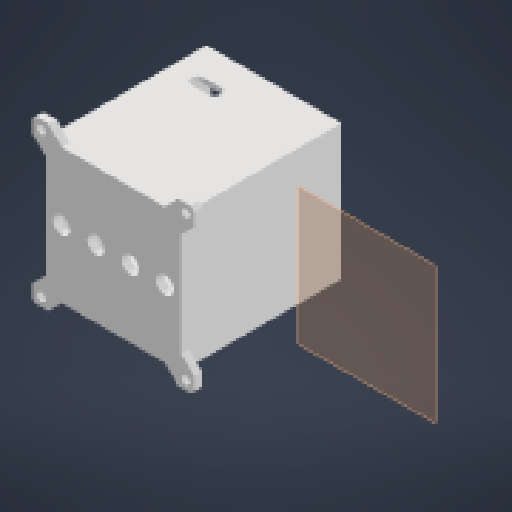
# Autodesk Inventor part: casing_1x1_lvl3
Saved by Autodesk Inventor 2024 (Build 280153000, 153)
## iProperties
Created: 2026-04-07
Part Number: casing_1x1_lvl3
Material: Generic
Document SubType Name: Modeling
Designer: schar
Density: 1 g/cm^3
Appearance: Default
Author: schar
Autodesk Inventor part; units mm, degrees
ref_plane "YZ Plane" through (0, 0, 0) normal (1, 0, 0) x (0, 1, 0)
ref_plane "XZ Plane" through (0, 0, 0) normal (0, 1, 0) x (-1, 0, 0)
ref_plane "XY Plane" through (0, 0, 0) normal (0, 0, 1) x (1, 0, 0)
sketch "Sketch1" plane through (0, 0, 0) normal (0, 0, 1) x (1, 0, 0)
  line L0 (51.6317, -54.9773) -> (91.6317, -54.9773) projected
  line L1 (94.6317, -57.9773) -> (94.5909, -98.4705) projected
  line L2 (48.6317, -97.9773) -> (48.6317, -57.9773) projected
  line L3 (91.6317, -100.9773) -> (51.6317, -100.9773) projected
  line L4 (48.6317, -77.9773) -> (94.6113, -78.2239)
  line L5 (71.6317, -54.9773) -> (71.6317, -100.9773)
  line L6 (48.5522, -54.8773) -> (94.7112, -54.8773)
  line L7 (94.7112, -54.8773) -> (94.7112, -101.0773)
  line L8 (94.7112, -101.0773) -> (48.5522, -101.0773)
  line L9 (48.5522, -101.0773) -> (48.5522, -54.8773)
  line L10 (48.5522, -54.8773) -> (94.7112, -101.0773) construction
  line L11 (94.7112, -54.8773) -> (48.5522, -101.0773) construction
  line L12 (46.6317, -52.9773) -> (96.6317, -52.9773)
  line L13 (96.6317, -52.9773) -> (96.6317, -102.9773)
  line L14 (96.6317, -102.9773) -> (46.6317, -102.9773)
  line L15 (46.6317, -102.9773) -> (46.6317, -52.9773)
  line L16 (46.6317, -52.9773) -> (96.6317, -102.9773) construction
  line L17 (96.6317, -52.9773) -> (46.6317, -102.9773) construction
  line L18 (36.6317, -42.9773) -> (106.6317, -42.9773)
  line L19 (106.6317, -42.9773) -> (106.6317, -112.9773)
  line L20 (106.6317, -112.9773) -> (36.6317, -112.9773)
  line L21 (36.6317, -112.9773) -> (36.6317, -42.9773)
  line L22 (36.6317, -42.9773) -> (106.6317, -112.9773) construction
  line L23 (106.6317, -42.9773) -> (36.6317, -112.9773) construction
  point P0 (0, 0)
  point P1 (71.6317, -77.9773)
  dimension "d0" = 46.159
  dimension "d1" = 46.2
  dimension "d2" = 50
  dimension "d3" = 50
  dimension "d4" = 70
  dimension "d5" = 70
  constraints: 40 end point, 11 midpoint, 6 parallel, 3 horizontal, 3 perpendicular
  measures "d0" distance of L7.end L8.end
  measures "d1" distance of L6.end L7.end
  measures "d2" distance of L13.end L14.end
  measures "d3" distance of L12.end L13.end
  measures "d4" distance of L19.end L20.end
  measures "d5" distance of L18.end L19.end
extrude "Extrusion1" add sketch "Sketch1" along normal blind 40 and the other way blind 30 contours L12 L13 L14 L15
ref_plane "Work Plane1" through (0, 0, 0) normal (0, 0, 1) x (1, 0, 0)
sketch "Sketch2" plane through (0, 0, 0) normal (0, 0, 1) x (1, 0, 0)
  arc A0 (94.6317, -57.9773) -> (91.6317, -54.9773) centre (91.6317, -57.9773) ccw projected
  line L0 (51.6317, -54.9773) -> (91.6317, -54.9773) projected
  arc A1 (51.6317, -54.9773) -> (48.6317, -57.9773) centre (51.6317, -57.9773) ccw projected
  line L1 (48.6317, -97.9773) -> (48.6317, -57.9773) projected
  arc A2 (48.6317, -97.9773) -> (51.6317, -100.9773) centre (51.6317, -97.9773) ccw projected
  line L2 (91.6317, -100.9773) -> (51.6317, -100.9773) projected
  arc A3 (91.6317, -100.9773) -> (94.5909, -98.4705) centre (91.6317, -97.9773) ccw projected
  line L3 (94.6317, -57.9773) -> (94.5909, -98.4705) projected
  circle A4 centre (51.6317, -97.9773) radius 1.1 projected
  circle A5 centre (56.1317, -83.4773) radius 1.725 projected
  circle A6 centre (62.4817, -82.2073) radius 0.45 projected
  circle A7 centre (65.0217, -80.9373) radius 0.45 projected
  circle A8 centre (62.4817, -79.6673) radius 0.45 projected
  circle A9 centre (65.0217, -78.3973) radius 0.45 projected
  circle A10 centre (72.1317, -96.7573) radius 0.5 projected
  circle A11 centre (72.1317, -94.2173) radius 0.5 projected
  circle A12 centre (72.1317, -91.6773) radius 0.5 projected
  circle A13 centre (72.1317, -89.1373) radius 0.5 projected
  circle A14 centre (79.1317, -89.9898) radius 0.4 projected
  circle A15 centre (91.6317, -97.9773) radius 1.1 projected
  circle A16 centre (86.7517, -89.9898) radius 0.4 projected
  circle A17 centre (72.1317, -86.5973) radius 0.5 projected
  circle A18 centre (72.1317, -84.0573) radius 0.5 projected
  circle A19 centre (72.1317, -81.5173) radius 0.5 projected
  circle A20 centre (72.1317, -78.9773) radius 0.5 projected
  circle A21 centre (78.5917, -81.7473) radius 0.45 projected
  circle A22 centre (78.5917, -79.2073) radius 0.45 projected
  circle A23 centre (81.1317, -80.4773) radius 0.45 projected
  circle A24 centre (87.4817, -83.0173) radius 1.725 projected
  circle A25 centre (56.1317, -72.0473) radius 1.725 projected
  circle A26 centre (62.4817, -77.1273) radius 0.45 projected
  circle A27 centre (65.0217, -75.8573) radius 0.45 projected
  circle A28 centre (62.4817, -74.5873) radius 0.45 projected
  circle A29 centre (65.0217, -73.3173) radius 0.45 projected
  arc A30 (55.0117, -62.6123) -> (55.6117, -62.6123) centre (55.3117, -62.6123) ccw projected
  line L4 (55.0117, -62.6123) -> (55.0117, -61.5123) projected
  arc A31 (55.6117, -61.5123) -> (55.0117, -61.5123) centre (55.3117, -61.5123) ccw projected
  line L5 (55.6117, -61.5123) -> (55.6117, -62.6123) projected
  circle A32 centre (51.6317, -57.9773) radius 1.1 projected
  arc A33 (55.0117, -58.1823) -> (55.6117, -58.1823) centre (55.3117, -58.1823) ccw projected
  line L6 (55.0117, -58.1823) -> (55.0117, -57.5823) projected
  arc A34 (55.6117, -57.5823) -> (55.0117, -57.5823) centre (55.3117, -57.5823) ccw projected
  line L7 (55.6117, -57.5823) -> (55.6117, -58.1823) projected
  circle A35 centre (56.7417, -61.5323) radius 0.325 projected
  circle A36 centre (62.5217, -61.5323) radius 0.325 projected
  arc A37 (63.6517, -62.6123) -> (64.2517, -62.6123) centre (63.9517, -62.6123) ccw projected
  line L8 (63.6517, -62.6123) -> (63.6517, -61.5123) projected
  arc A38 (64.2517, -61.5123) -> (63.6517, -61.5123) centre (63.9517, -61.5123) ccw projected
  line L9 (64.2517, -61.5123) -> (64.2517, -62.6123) projected
  arc A39 (63.6517, -58.1823) -> (64.2517, -58.1823) centre (63.9517, -58.1823) ccw projected
  line L10 (63.6517, -58.1823) -> (63.6517, -57.5823) projected
  arc A40 (64.2517, -57.5823) -> (63.6517, -57.5823) centre (63.9517, -57.5823) ccw projected
  line L11 (64.2517, -57.5823) -> (64.2517, -58.1823) projected
  circle A41 centre (72.1317, -76.4373) radius 0.5 projected
  circle A42 centre (72.1317, -73.8973) radius 0.5 projected
  circle A43 centre (78.5917, -76.6673) radius 0.45 projected
  circle A44 centre (81.1317, -77.9373) radius 0.45 projected
  circle A45 centre (81.1317, -75.3973) radius 0.45 projected
  circle A46 centre (78.5917, -74.1273) radius 0.45 projected
  circle A47 centre (81.1317, -72.8573) radius 0.45 projected
  circle A48 centre (72.1317, -71.3573) radius 0.5 projected
  circle A49 centre (72.1317, -68.8173) radius 0.5 projected
  circle A50 centre (87.4817, -71.5873) radius 1.725 projected
  circle A51 centre (72.1317, -66.2773) radius 0.5 projected
  circle A52 centre (72.1317, -63.7373) radius 0.5 projected
  circle A53 centre (72.1317, -61.1973) radius 0.5 projected
  circle A54 centre (72.1317, -58.6573) radius 0.5 projected
  circle A55 centre (91.6317, -57.9773) radius 1.1 projected
  circle A56 centre (51.6317, -57.9773) radius 1.1
  circle A57 centre (91.6317, -57.9773) radius 1.1
  circle A58 centre (91.6317, -97.9773) radius 1.1
  circle A59 centre (51.6317, -97.9773) radius 1.1
  line L12 (48.5522, -101.0773) -> (94.7112, -101.0773) projected
  line L13 (48.5522, -101.0773) -> (53.5522, -101.0773)
  line L14 (53.5522, -101.0773) -> (53.5522, -96.0773)
  line L15 (53.5522, -96.0773) -> (48.5522, -96.0773)
  line L16 (48.5522, -96.0773) -> (48.5522, -101.0773)
  line L17 (94.7112, -101.0773) -> (89.7112, -101.0773)
  line L18 (89.7112, -101.0773) -> (89.7112, -96.0773)
  line L19 (89.7112, -96.0773) -> (94.7112, -96.0773)
  line L20 (94.7112, -96.0773) -> (94.7112, -101.0773)
  line L21 (94.7112, -54.8773) -> (89.7112, -54.8773)
  line L22 (89.7112, -54.8773) -> (89.7112, -59.8773)
  line L23 (89.7112, -59.8773) -> (94.7112, -59.8773)
  line L24 (94.7112, -59.8773) -> (94.7112, -54.8773)
  line L25 (48.5522, -54.8773) -> (53.5522, -54.8773)
  line L26 (53.5522, -54.8773) -> (53.5522, -59.8773)
  line L27 (53.5522, -59.8773) -> (48.5522, -59.8773)
  line L28 (48.5522, -59.8773) -> (48.5522, -54.8773)
  point P0 (0, 0)
  point P1 (99.5, 70)
  point P2 (102.5, 113)
  point P3 (145.4592, 110.4932)
  dimension "d10" = 5
  dimension "d11" = 5
  dimension "d12" = 5
  dimension "d13" = 5
  dimension "d14" = 5
  dimension "d15" = 5
  dimension "d16" = 5
  dimension "d17" = 5
  constraints: 32 end point, 8 parallel, 4 centre point, 4 coincident, 4 concentric, 4 horizontal, 4 perpendicular, 1 point on line
  measures "d10" distance of L15.end L14.end
  measures "d11" distance of L14.end L13.end
  measures "d12" distance of L18.end L19.end
  measures "d13" distance of L17.end L18.end
  measures "d14" distance of L23.end L22.end
  measures "d15" distance of L22.end L21.end
  measures "d16" distance of L26.end L27.end
  measures "d17" distance of L25.end L26.end
extrude "Extrusion2" add sketch "Sketch2" along normal blind 10 contours L3 L23 L22 L0 A0 | A0 L0 L22 L21 L24 L23 L3 | L19 L20 L12 L18 L2 A3 L3 | L3 A3 L2 L18 L19 | L26 L27 L1 A1 L0 | L0 A1 L1 L27 L28 L25 L26 | L14 L12 L16 L15 L1 A2 L2 | L2 A2 L1 L15 L14
sketch "Sketch5" plane through (0, 0, 40) normal (0, 0, 1) x (1, 0, 0)
  line L0 (96.6317, -52.9773) -> (46.6317, -52.9773) projected
  line L1 (71.6317, -52.9773) -> (71.6317, -102.9773)
  line L2 (46.6317, -102.9773) -> (96.6317, -102.9773) projected
  line L3 (96.6317, -102.9773) -> (96.6317, -52.9773) projected
  line L4 (96.6317, -77.9773) -> (46.6317, -77.9773)
  line L5 (46.6317, -102.9773) -> (46.6317, -52.9773) projected
  line L6 (41.6317, -47.9773) -> (101.6317, -47.9773)
  line L7 (101.6317, -47.9773) -> (101.6317, -107.9773)
  line L8 (101.6317, -107.9773) -> (41.6317, -107.9773)
  line L9 (41.6317, -107.9773) -> (41.6317, -47.9773)
  line L10 (41.6317, -47.9773) -> (101.6317, -107.9773) construction
  line L11 (101.6317, -47.9773) -> (41.6317, -107.9773) construction
  line L12 (96.6317, -52.9773) -> (96.6317, -58.9773)
  line L13 (96.6317, -52.9773) -> (90.6317, -52.9773)
  line L14 (90.6317, -52.9773) -> (95.6317, -47.9773)
  line L15 (95.6317, -47.9773) -> (101.6317, -47.9773)
  line L16 (101.6317, -47.9773) -> (101.6317, -53.9773)
  line L17 (101.6317, -53.9773) -> (96.6317, -58.9773)
  line L18 (96.6317, -52.9773) -> (98.3995, -51.2096)
  circle A0 centre (98.3995, -51.2096) radius 1.5
  circle A1 centre (44.8639, -51.2096) radius 1.5
  line L19 (47.6317, -47.9773) -> (52.6317, -52.9773)
  line L20 (46.6317, -52.9773) -> (52.6317, -52.9773)
  line L21 (46.6317, -52.9773) -> (46.6317, -58.9773)
  line L22 (46.6317, -58.9773) -> (41.6317, -53.9773)
  line L23 (41.6317, -47.9773) -> (101.6317, -107.9773) construction
  line L24 (46.6317, -52.9773) -> (44.8639, -51.2096)
  circle A2 centre (44.8639, -104.7451) radius 1.5
  line L25 (41.6317, -101.9773) -> (46.6317, -96.9773)
  line L26 (46.6317, -102.9773) -> (46.6317, -96.9773)
  line L27 (46.6317, -102.9773) -> (52.6317, -102.9773)
  line L28 (52.6317, -102.9773) -> (47.6317, -107.9773)
  line L29 (41.6317, -107.9773) -> (101.6317, -47.9773) construction
  line L30 (46.6317, -102.9773) -> (44.8639, -104.7451)
  circle A3 centre (98.3995, -104.7451) radius 1.5
  line L31 (95.6317, -107.9773) -> (90.6317, -102.9773)
  line L32 (96.6317, -102.9773) -> (90.6317, -102.9773)
  line L33 (96.6317, -102.9773) -> (96.6317, -96.9773)
  line L34 (96.6317, -96.9773) -> (101.6317, -101.9773)
  line L35 (101.6317, -107.9773) -> (41.6317, -47.9773) construction
  line L36 (96.6317, -102.9773) -> (98.3995, -104.7451)
  point P0 (0, 0)
  point P1 (71.6317, -77.9773)
  point P2 (71.6317, -77.9773)
  point P3 (71.6317, -77.9773)
  point P4 (71.6317, -77.9773)
  point P5 (52.6317, -52.9773)
  point P6 (47.6317, -47.9773)
  point P7 (41.6317, -53.9773)
  point P8 (46.6317, -58.9773)
  point P9 (46.6317, -96.9773)
  point P10 (41.6317, -101.9773)
  point P11 (47.6317, -107.9773)
  point P12 (52.6317, -102.9773)
  point P13 (90.6317, -102.9773)
  point P14 (95.6317, -107.9773)
  point P15 (101.6317, -101.9773)
  point P16 (96.6317, -96.9773)
  dimension "d35" = 60
  dimension "d36" = 60
  dimension "d37" = 6
  dimension "d38" = 6
  dimension "d39" = 2.5
  dimension "d40" = 45
  dimension "d41" = 3
  dimension "d44" = 360
  constraints: 66 end point, 8 point on line, 7 midpoint, 6 coincident, 4 centre point, 4 parallel, 1 horizontal, 1 perpendicular, 67 other
  measures "d35" distance of L7.end L8.end
  measures "d36" distance of L6.end L7.end
  measures "d37" distance of L0.start L12.end
  measures "d38" distance of L0.start L13.end
  measures "d39" distance of L0.start L18.end
  measures "d40" angle of L17 L12
  measures "d41" diameter of A0
extrude "Extrusion5" add sketch "Sketch5" along normal blind 3 contours L3 L4 L1 L0 | L0 L14 L6 L7 L17 L3 | L1 L4 L5 L0 | L3 L2 L1 L4 | L0 L5 L22 L9 L6 L19 | L1 L2 L5 L4 | L34 L7 L8 L31 L2 L3 | L28 L8 L9 L25 L5 L2
sketch "Sketch6" plane through (0, 0, -30) normal (0, 0, -1) x (-1, 0, 0)
  line L0 (-96.6317, -102.9773) -> (-46.6317, -102.9773) projected
  line L1 (-46.6317, -102.9773) -> (-46.6317, -52.9773) projected
  line L2 (-46.6317, -52.9773) -> (-96.6317, -52.9773) projected
  line L3 (-96.6317, -52.9773) -> (-96.6317, -102.9773) projected
  line L4 (-94.7112, -54.8773) -> (-48.5522, -54.8773) projected
  line L5 (-48.5522, -54.8773) -> (-48.5522, -101.0773) projected
  line L6 (-48.5522, -101.0773) -> (-94.7112, -101.0773) projected
  line L7 (-94.7112, -101.0773) -> (-94.7112, -54.8773) projected
  line L8 (-96.6317, -52.9773) -> (-46.6317, -52.9773)
  line L9 (-46.6317, -52.9773) -> (-46.6317, -102.9773)
  line L10 (-46.6317, -102.9773) -> (-96.6317, -102.9773)
  line L11 (-96.6317, -102.9773) -> (-96.6317, -52.9773)
  point P0 (0, 0)
  constraints: 8 end point, 2 parallel, 1 horizontal, 1 perpendicular
ref_plane "Work Plane2" through (100.7, -97.28, -17.595) normal (0, 0, -1) x (0, 1, 0)
ref_plane "Work Plane3" through (99.4205, -113.1, -16.51) normal (0, 0, -1) x (0, 1, 0)
extrude "Extrusion6" cut sketch "Sketch6" against normal up to surface (13.49 mm away) contours L3 L2 L1 L0 | L4 L5 L6 L7
sketch "Sketch7" plane through (0, 0, 43) normal (0, 0, 1) x (1, 0, 0)
  line L0 (48.5522, -101.0773) -> (48.5522, -54.8773) projected
  line L1 (48.5522, -77.9773) -> (94.7112, -77.9773)
  line L2 (94.7112, -54.8773) -> (94.7112, -101.0773) projected
  line L3 (71.6317, -77.9773) -> (134.04, -77.9773)
  line L4 (48.5522, -77.9773) -> (52.5522, -77.9773)
  line L5 (94.7112, -77.9773) -> (90.7112, -77.9773)
  circle A0 centre (52.5522, -77.9773) radius 3.175
  circle A1 centre (90.7112, -77.9773) radius 3.175
  line L6 (55.7272, -77.9773) -> (117.1985, -77.9773)
  line L7 (117.1985, -77.9773) -> (127.8015, -77.9773)
  line L8 (52.5522, -77.9773) -> (65.2719, -77.9773)
  line L9 (65.2719, -77.9773) -> (77.9914, -77.9773)
  circle A2 centre (65.2719, -77.9773) radius 3.175
  circle A3 centre (77.9914, -77.9773) radius 3.175
  point P0 (0, 0)
  dimension "d56" = 6.35
  dimension "d54" = 4
  dimension "d55" = 4
  dimension "d57" = 6.35
  dimension "d60" = 12.7197
  dimension "d61" = 12.7195
  dimension "d62" = 6.35
  dimension "d63" = 6.35
  constraints: 16 end point, 8 point on line, 4 coincident, 3 centre point, 3 midpoint, 1 horizontal alignment, 2 other
  measures "d54" distance of L1.start L4.end
  measures "d55" distance of L1.end L5.end
  measures "d57" diameter of A1
  measures "d60" distance of L8.start L8.end
  measures "d61" distance of L8.end L9.end
  measures "d62" diameter of A2
  measures "d63" diameter of A3
extrude "Extrusion7" cut sketch "Sketch7" against normal blind 10
fillet "Fillet1" radius 2 4 edges at (41.6317, -47.9773, 41.5) (101.6317, -47.9773, 41.5) (101.6317, -107.9773, 41.5) (41.6317, -107.9773, 41.5)
sketch "Sketch8" plane through (52.6317, -52.9773, 43) normal (0, 1, 0) x (1, 0, 0)
  line L0 (10.19, 47.82) -> (3.81, 47.82) projected
  arc A0 (11.47, 46.54) -> (10.19, 47.82) centre (10.19, 46.54) ccw projected
  arc A1 (10.19, 44.66) -> (11.47, 45.94) centre (10.19, 45.94) ccw projected
  arc A2 (3.81, 47.82) -> (2.53, 46.54) centre (3.81, 46.54) ccw projected
  arc A3 (3.81, 47.82) -> (2.53, 46.54) centre (3.81, 46.54) ccw projected
  line L1 (2.53, 46.54) -> (2.53, 45.94) projected
  arc A4 (2.53, 45.94) -> (3.81, 44.66) centre (3.81, 45.94) ccw projected
  line L2 (3.81, 44.66) -> (6.495, 44.66) projected
  line L3 (6.495, 44.66) -> (6.495, 44.86) projected
  line L4 (6.495, 44.86) -> (3.81, 44.86) projected
  arc A5 (2.73, 45.94) -> (3.81, 44.86) centre (3.81, 45.94) ccw projected
  line L5 (2.73, 46.54) -> (2.73, 45.94) projected
  arc A6 (3.81, 47.62) -> (2.73, 46.54) centre (3.81, 46.54) ccw projected
  line L6 (3.81, 47.62) -> (10.19, 47.62) projected
  arc A7 (11.27, 46.54) -> (10.19, 47.62) centre (10.19, 46.54) ccw projected
  line L7 (11.27, 45.94) -> (11.27, 46.54) projected
  arc A8 (10.19, 44.86) -> (11.27, 45.94) centre (10.19, 45.94) ccw projected
  line L8 (6.505, 44.86) -> (10.19, 44.86) projected
  line L9 (6.505, 44.86) -> (6.505, 44.66) projected
  line L10 (6.505, 44.66) -> (10.19, 44.66) projected
  arc A9 (10.19, 44.66) -> (11.47, 45.94) centre (10.19, 45.94) ccw projected
  line L11 (11.47, 45.94) -> (11.47, 46.54) projected
  arc A10 (11.47, 46.54) -> (10.19, 47.82) centre (10.19, 46.54) ccw projected
  line L12 (10.19, 47.82) -> (3.81, 47.82) projected
  line L13 (3.75, 48.49) -> (10.25, 48.49)
  line L14 (12.25, 46.49) -> (12.25, 45.99)
  line L15 (10.25, 43.99) -> (3.75, 43.99)
  line L16 (1.75, 45.99) -> (1.75, 46.49)
  line L17 (1.75, 48.49) -> (12.25, 43.99) construction
  line L18 (12.25, 48.49) -> (1.75, 43.99) construction
  arc A11 (3.75, 48.49) -> (1.75, 46.49) centre (3.75, 46.49) ccw
  arc A12 (12.25, 46.49) -> (10.25, 48.49) centre (10.25, 46.49) ccw
  arc A13 (10.25, 43.99) -> (12.25, 45.99) centre (10.25, 45.99) ccw
  arc A14 (1.75, 45.99) -> (3.75, 43.99) centre (3.75, 45.99) ccw
  point P0 (-52.6317, 43)
  point P1 (7, 46.24)
  dimension "d67" = 10.5
  dimension "d68" = 4.5
  dimension "d69" = 2
  constraints: 12 end point, 8 point on circle, 8 point on line, 8 tangent, 4 centre point, 3 equal radius, 2 midpoint, 2 parallel, 1 horizontal, 1 perpendicular
  measures "d67" distance of L17.end L18.end
  measures "d68" distance of L18.start L17.end
  measures "d69" radius of A11
extrude "Extrusion8" cut sketch "Sketch8" against normal up to surface (1.9 mm away) contours A0 L11 A1 L10 L9 L8 A8 L7 A7 L6 A6 L5 A5 L4 L3 L2 A4 L1 A2 L0 | L13 A12 L14 A13 L15 A14 L16 A11
fillet "Fillet2" radius 1.5 8 edges at (54.9675, -52.9773, -1.5758) (54.3817, -52.9773, -3.24) (54.9675, -52.9773, -4.9042) (59.6317, -52.9773, -5.49) (64.2959, -52.9773, -4.9042) (64.8817, -52.9773, -3.24) (64.2959, -52.9773, -1.5758) (59.6317, -52.9773, -0.99) inverted yes
body "Solid1"
